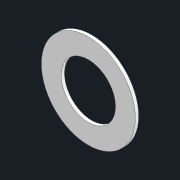
# Autodesk Inventor part: unit-spapcer1
Saved by Autodesk Inventor 2021 (Build 250183000, 183)
## iProperties
Created: 2021-02-03
Part Number: unit-spapcer1
Material: ABS プラスチック
Document SubType Name: Modeling
Designer: Yuta Kage
Mass: 0.025625 g
Surface Area: 1.22145 cm^2
Volume: 0.0241746 cm^3
Density: 1.06 g/cm^3
Appearance: 滑らか - 白
Description: 3Dプリント
Author: Yuta Kage
Autodesk Inventor part; units mm, degrees
ref_plane "YZ Plane" through (0, 0, 0) normal (1, 0, 0) x (0, 1, 0)
ref_plane "XZ Plane" through (0, 0, 0) normal (0, 1, 0) x (-1, 0, 0)
ref_plane "XY Plane" through (0, 0, 0) normal (0, 0, 1) x (1, 0, 0)
sketch "スケッチ1" plane through (0, 0, 0) normal (0, 0, 1) x (1, 0, 0)
  circle A0 centre (0, 0) radius 4.05
  circle A1 centre (0, 0) radius 7
  dimension "d0" = 8.1
  dimension "d1" = 14
  constraints: 2 centre point, 2 coincident
  measures "d0" diameter of A0
  measures "d1" diameter of A1
extrude "押し出し1" add sketch "スケッチ1" along normal blind 0.5
